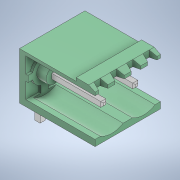
# Autodesk Inventor part: plugin_maleblock
Saved by Autodesk Inventor 2020 (Build 240168000, 168)
## iProperties
Created: 2019-08-19
Part Number: plugin_maleblock
Material: Generic
Document SubType Name: Modeling
Designer: SENSE IT OUT
Density: 1 g/cm^3
Appearance: Default
Mass: 0.267438 g
Surface Area: 8.31838 cm^2
Volume: 0.267438 cm^3
Author: SENSE IT OUT
Autodesk Inventor part; units mm, degrees
ref_plane "YZ Plane" through (0, 0, 0) normal (1, 0, 0) x (0, 1, 0)
ref_plane "XZ Plane" through (0, 0, 0) normal (0, 1, 0) x (-1, 0, 0)
ref_plane "XY Plane" through (0, 0, 0) normal (0, 0, 1) x (1, 0, 0)
sketch "Sketch1" plane through (0, 0, 0) normal (0, 0, 1) x (1, 0, 0)
  line L0 (0, 0) -> (12, 0)
  line L1 (9, 7.5) -> (0, 7.5)
  line L2 (0, 7.5) -> (0, 0)
  line L3 (1, 1) -> (11, 1)
  line L4 (1, 6.5) -> (1, 1)
  line L5 (11, 1) -> (12, 1)
  line L6 (12, 1) -> (12, 0)
  line L7 (12, 7.5) -> (12, 7)
  line L8 (12, 7) -> (1, 7)
  line L9 (1, 6.5) -> (1, 7)
  line L10 (11, 8) -> (9, 8)
  line L11 (9, 8) -> (9, 7.5)
  line L12 (12, 7.5) -> (11, 8)
  dimension "d0" = 7.5
  dimension "d1" = 1
  dimension "d3" = 10
  dimension "d4" = 1
  dimension "d5" = 1
  dimension "d6" = 0.5
  dimension "d7" = 11
  dimension "d10" = 0.5
  dimension "d11" = 11
  dimension "d12" = 0.5
  dimension "d14" = 1
  dimension "d15" = 3
  dimension "d16" = 1
  constraints: 26 end point, 4 perpendicular, 1 horizontal, 1 parallel, 1 vertical
  measures "d0" distance between parallel lines of L0 L1
  measures "d1" distance between parallel lines of L2 L4
  measures "d3" distance of L3.start L3.end
  measures "d4" distance of L3.end L5.end
  measures "d5" distance of L5.end L0.end
  measures "d6" distance of L7.start L7.end
  measures "d7" distance of L7.end L8.end
  measures "d10" distance of L10.end L1.start
  measures "d11" distance between parallel lines of L4 L6
  measures "d12" distance from line of L8 L12.start
  measures "d14" distance from line of L7 L10.start
  measures "d15" distance between parallel lines of L7 L11
  measures "d16" distance between parallel lines of L8 L10
extrude "Extrusion1" add sketch "Sketch1" along normal blind 10.4
sketch "Sketch2" plane through (1, 1, 0) normal (1, 0, 0) x (0, 0, -1)
  circle A0 centre (-7.74, 3) radius 1.27
  circle A1 centre (-2.66, 3) radius 1.27
  line L0 (0, 0) -> (0, 6) projected
  line L1 (0, 0) -> (-10.4, 0) projected
  circle A2 centre (-7.74, 3) radius 2
  circle A3 centre (-2.66, 3) radius 2
  line L2 (-10.4, 0) -> (-10.4, 6) projected
  line L3 (0, 6) -> (-10.4, 6) projected
  line L4 (-7.14, 0) -> (-7.14, 1.0921)
  line L5 (-7.14, 4.9079) -> (-7.14, 6)
  line L6 (-8.34, 6) -> (-8.34, 4.9079)
  line L7 (-8.34, 1.0921) -> (-8.34, 0)
  line L8 (-2.06, 0) -> (-2.06, 1.0921)
  line L9 (-2.06, 4.9079) -> (-2.06, 6)
  line L10 (-3.26, 6) -> (-3.26, 4.9079)
  line L11 (-3.26, 1.0921) -> (-3.26, 0)
  line L12 (-0.7235, 3.5) -> (0, 3.5)
  line L13 (0, 2.5) -> (-0.7235, 2.5)
  line L14 (-5.8035, 3.5) -> (-4.5965, 3.5)
  line L15 (-4.5965, 2.5) -> (-5.8035, 2.5)
  line L16 (-9.6765, 2.5) -> (-10.4, 2.5)
  line L17 (-10.4, 3.5) -> (-9.6765, 3.5)
  point P0 (0, -1)
  dimension "d25" = 4
  dimension "d26" = 4
  dimension "d19" = 5.08
  dimension "d20" = 2.66
  dimension "d21" = 0
  dimension "d22" = 3
  dimension "d23" = 2.54
  dimension "d24" = 2.54
  constraints: 28 end point, 12 perpendicular, 10 point on line, 9 parallel, 3 horizontal, 2 centre point, 2 coincident, 20 other
  measures "d19" distance of A1.centre A0.centre
  measures "d20" distance from line of L0 A1.centre
  measures "d21" vertical distance of A0.centre A1.centre
  measures "d22" distance from line of L1 A1.centre
  measures "d23" diameter of A0
  measures "d24" diameter of A1
extrude "Extrusion2" add sketch "Sketch2" along normal blind 0.35 contours L13 A3 L12 L0 | L1 L11 A3 L8 | A3 | L1 L7 A2 L4 | L9 A3 L10 L3 | A2 | L15 A2 L14 A3 | L5 A2 L6 L3 | L2 L17 A2 L16
sketch "Sketch3" plane through (1.35, 1, 0) normal (1, 0, 0) x (0, 0, -1)
  circle A0 centre (-7.74, 3) radius 1.27 projected
  circle A1 centre (-7.74, 3) radius 1.27
  circle A2 centre (-7.74, 3) radius 2
  circle A3 centre (-2.66, 3) radius 1.27 projected
  circle A4 centre (-2.66, 3) radius 1.27
  circle A5 centre (-2.66, 3) radius 2
  circle A6 centre (-7.74, 3) radius 1.27
  circle A7 centre (-7.74, 3) radius 0.75
  circle A8 centre (-2.66, 3) radius 1.27
  circle A9 centre (-2.66, 3) radius 0.75
  point P0 (0, -1)
  dimension "d49" = 1.5
  dimension "d50" = 1.5
  constraints: 8 centre point, 8 coincident, 1 concentric
  measures "d49" diameter of A7
  measures "d50" diameter of A9
extrude "Extrusion3" add sketch "Sketch3" along normal blind 1.5 contours A0 | A3 | A7 | A9
sketch "Sketch5" plane through (2.85, 4, 7.74) normal (1, 0, 0) x (0, 0, -1)
  line L0 (4.68, 0.4) -> (5.48, 0.4)
  line L1 (5.48, 0.4) -> (5.48, -0.4)
  line L2 (5.48, -0.4) -> (4.68, -0.4)
  line L3 (4.68, -0.4) -> (4.68, 0.4)
  line L4 (-0.4, 0.4) -> (0.4, 0.4)
  line L5 (0.4, 0.4) -> (0.4, -0.4)
  line L6 (0.4, -0.4) -> (-0.4, -0.4)
  line L7 (-0.4, -0.4) -> (-0.4, 0.4)
  circle A0 centre (5.08, 0) radius 1.27 projected
  circle A1 centre (0, 0) radius 1.27 projected
  point P0 (7.74, -4)
  dimension "d51" = 0.4
  dimension "d52" = 0.8
  dimension "d53" = 0.8
  dimension "d54" = 0.4
  dimension "d55" = 0.8
  dimension "d56" = 0.8
  dimension "d57" = 0.4
  constraints: 16 end point, 4 parallel, 2 horizontal, 2 perpendicular, 1 point on line
  measures "d51" distance from line of A0.centre L0
  measures "d52" distance of L0.start L0.end
  measures "d53" distance of L2.end L0.start
  measures "d54" distance from line of A0.centre L3
  measures "d55" distance of L4.start L4.end
  measures "d56" distance of L6.end L4.start
  measures "d57" distance from line of A1.centre L7
extrude "Extrusion5" add sketch "Sketch5" along normal blind 8 contours L0 L1 L2 L3 | L4 L5 L6 L7
chamfer "Chamfer2" distance 0.2 angle 45 8 edges at (10.85, 4.4, 7.74) (10.85, 4.4, 2.66) (10.85, 4, 2.26) (10.85, 4, 3.06) (10.85, 3.6, 2.66) (10.85, 4, 8.14) (10.85, 4, 7.34) (10.85, 3.6, 7.74)
sketch "Sketch6" plane through (9, 8, 0) normal (0, 1, 0) x (1, 0, 0)
  line L0 (3, 0) -> (3, -10.4) projected
  line L1 (2, 0) -> (2, -10.4) projected
  line L2 (3, -0.55) -> (2, -0.55)
  line L3 (2, -0.55) -> (2, -2.05)
  line L4 (2, -2.05) -> (3, -2.05)
  line L5 (3, -2.05) -> (3, -0.55)
  line L6 (3, -0.55) -> (2, -0.8)
  line L7 (3, -2.05) -> (2, -1.8)
  line L8 (3, 0) -> (2, 0) projected
  point P0 (-9, 0)
  point P1 (2, -1.8)
  point P2 (3, -2.05)
  dimension "d69" = 1.5
  dimension "d70" = 1
  dimension "d71" = 0.25
  dimension "d72" = 0.55
  constraints: 12 end point, 4 point on line, 2 parallel, 1 horizontal, 1 perpendicular
  measures "d69" distance between parallel lines of L4 L2
  measures "d70" distance of L7.end L6.end
  measures "d71" distance from line of L2 L6.end
  measures "d72" distance between parallel lines of L8 L2
extrude "Extrusion6" cut sketch "Sketch6" against normal blind 5 contours L0 L7 L1 L6
pattern_linear "Rectangular Pattern1" count 4 spacing 2.6 along (0, 0, 1) of "Extrusion6"
sketch "Sketch7" plane through (12, 0, 0) normal (1, 0, 0) x (0, 0, -1)
  circle A0 centre (-7.74, 4) radius 1.27 projected
  arc A1 (-9.5428, 1) -> (-5.9372, 1) centre (-7.74, 4) ccw
  arc A2 (-4.4628, 1) -> (-0.8572, 1) centre (-2.66, 4) ccw
  circle A3 centre (-2.66, 4) radius 1.27 projected
  line L0 (0, 1) -> (-10.4, 1) projected
  line L1 (-5.9372, 1) -> (-4.4628, 1)
  line L2 (-8.34, 1) -> (-10.4, 1) projected
  line L3 (-9.5428, 1) -> (-10.4, 1)
  line L4 (-10.4, 1) -> (0, 1)
  point P0 (0, 0)
  dimension "d78" = 7
  dimension "d79" = 7
  constraints: 6 end point, 4 point on circle, 4 point on line, 2 centre point, 2 collinear, 1 coincident, 1 concentric
  measures "d78" diameter of A1
  measures "d79" diameter of A2
extrude "Extrusion7" cut sketch "Sketch7" against normal blind 10.65 contours L0 A1 | L0 A2
sketch "Sketch8" plane through (0, 0, 0) normal (0, -1, 0) x (1, 0, 0)
  line L0 (1, 2.26) -> (-0.413, 2.26)
  line L1 (-0.413, 2.26) -> (-0.413, 3.06)
  line L2 (-0.413, 3.06) -> (1, 3.06)
  line L3 (1, 3.06) -> (1, 2.26)
  line L4 (1, 7.34) -> (-0.9223, 7.34)
  line L5 (-0.9223, 7.34) -> (-0.9223, 8.14)
  line L6 (-0.9223, 8.14) -> (1, 8.14)
  line L7 (1, 8.14) -> (1, 7.34)
  line L8 (0, 0) -> (0, 10.4) projected
  line L9 (0, 0) -> (12, 0) projected
  line L10 (0, 10.4) -> (12, 10.4) projected
  line L11 (2.85, 8.14) -> (10.65, 8.14) projected
  line L12 (2.85, 2.26) -> (10.65, 2.26) projected
  point P0 (1, 10.4)
  dimension "d83" = 1
  dimension "d84" = 0.8
  dimension "d85" = 0.8
  dimension "d86" = 2.26
  dimension "d87" = 2.26
  dimension "d88" = 2.26
  dimension "d89" = 2.26
  constraints: 16 end point, 4 parallel, 2 horizontal, 1 perpendicular
  measures "d83" distance between parallel lines of L8 L7
  measures "d84" distance between parallel lines of L2 L0
  measures "d85" distance between parallel lines of L6 L4
  measures "d86" distance between parallel lines of L9 L0
  measures "d87" distance between parallel lines of L6 L10
  measures "d88" distance from line of point (1, 10.4) L11
  measures "d89" distance between parallel lines of L9 L12
extrude "Extrusion8" cut sketch "Sketch8" against normal blind 4.5
sketch "Sketch10" plane through (1, 0, 2.26) normal (-1, 0, 0) x (0, 0, 1)
  line L0 (0, 4.4) -> (0.8, 4.4)
  line L1 (0.8, 4.4) -> (0.8, -3.6)
  line L2 (0.8, -3.6) -> (0, -3.6)
  line L3 (0, -3.6) -> (0, 4.4)
  line L4 (5.08, 4.4) -> (5.88, 4.4)
  line L5 (5.88, 4.4) -> (5.88, -3.6)
  line L6 (5.88, -3.6) -> (5.08, -3.6)
  line L7 (5.08, -3.6) -> (5.08, 4.4)
  line L8 (0.8, 4.5) -> (0.8, 0) projected
  line L9 (5.08, 0) -> (5.08, 4.5) projected
  line L10 (0, 4.5) -> (0.8, 4.5) projected
  arc A0 (0.8, 2.7946) -> (0, 2.7946) centre (0.4, 4) ccw projected
  arc A1 (5.88, 2.7946) -> (5.08, 2.7946) centre (5.48, 4) ccw projected
  point P0 (-2.26, 0)
  dimension "d92" = 0.8
  dimension "d93" = 0.8
  dimension "d96" = 8
  dimension "d101" = 0.4
  dimension "d102" = 0.4
  dimension "d103" = 0.4
  dimension "d106" = 8
  constraints: 16 end point, 4 parallel, 2 horizontal, 2 perpendicular, 1 point on line
  measures "d92" distance of L5.end L6.end
  measures "d93" distance of L1.end L2.end
  measures "d96" distance of L2.end L0.start
  measures "d101" distance from line of L7 A1.centre
  measures "d102" distance from line of L0 A0.centre
  measures "d103" distance from line of L3 A0.centre
  measures "d106" distance of L6.end L4.start
extrude "Extrusion9" add sketch "Sketch10" along normal blind 0.8 contours L0 L1 L2 L3 | L4 L5 L6 L7
sketch "Sketch11" plane through (1, 1, 10.4) normal (1, 0, 0) x (0, 0, -1)
  point P0 (10.4, -1)
chamfer "Chamfer3" distance 0.2 angle 45 8 edges at (0.6, -3.6, 8.14) (0.2, -3.6, 7.74) (0.6, -3.6, 7.34) (1, -3.6, 7.74) (0.2, -3.6, 2.66) (0.6, -3.6, 2.26) (0.6, -3.6, 3.06) (1, -3.6, 2.66)
fillet "Fillet1" radius 0.2 2 edges at (0.2, 4.4, 2.66) (0.2, 4.4, 7.74)
sketch "Sketch12" plane through (0, 0, 0) normal (-1, 0, 0) x (0, 0, 1)
  line L0 (1.91, 7) -> (3.41, 7)
  line L1 (3.41, 7) -> (3.41, 0)
  line L2 (1.91, 0) -> (1.91, 7)
  line L3 (6.99, 7) -> (8.49, 7)
  line L4 (8.49, 7) -> (8.49, 0)
  line L5 (6.99, 0) -> (6.99, 7)
  line L6 (8.14, 0) -> (10.4, 0) projected
  line L7 (3.06, 0) -> (7.34, 0) projected
  line L8 (0, 7.5) -> (10.4, 7.5) projected
  line L9 (3.06, -3.4) -> (3.06, 0) projected
  line L10 (8.14, 4.5) -> (8.14, 0) projected
  line L11 (2.26, 0) -> (2.26, 4.5) projected
  line L12 (0, 0) -> (2.26, 0) projected
  line L13 (2.26, 0) -> (2.26, -3.4) projected
  line L14 (2.26, 4.4) -> (3.06, 4.4) projected
  line L15 (2.26, 0) -> (3.06, 0)
  line L16 (3.06, 0) -> (3.06, 4.4)
  line L17 (3.06, 4.4) -> (2.26, 4.4)
  line L18 (2.26, 4.4) -> (2.26, 0)
  line L19 (7.34, 4.4) -> (8.14, 4.4) projected
  line L20 (8.14, 0) -> (8.14, 4.4)
  line L21 (8.14, 4.4) -> (7.34, 4.4)
  line L22 (7.34, 4.4) -> (7.34, 0)
  line L23 (3.41, 0) -> (3.06, 0)
  line L24 (2.26, 0) -> (1.91, 0)
  line L25 (8.49, 0) -> (8.14, 0)
  line L26 (7.34, 0) -> (6.99, 0)
  point P0 (3.41, 0)
  dimension "d111" = 1.5
  dimension "d112" = 1.5
  dimension "d115" = 0.5
  dimension "d116" = 0.5
  dimension "d117" = 0.35
  dimension "d118" = 0.35
  constraints: 35 end point, 9 parallel, 3 horizontal, 3 perpendicular
  measures "d111" distance between parallel lines of L1 L2
  measures "d112" distance between parallel lines of L4 L5
  measures "d115" distance between parallel lines of L8 L0
  measures "d116" distance between parallel lines of L3 L8
  measures "d117" distance between parallel lines of L9 L1
  measures "d118" distance between parallel lines of L10 L4
extrude "Extrusion10" cut sketch "Sketch12" against normal blind 0.1 contours L5 L3 L4 L6 L10 L19 L22 L7 | L0 L1 L7 L16 L14 L11 L12 L2
sketch "Sketch13" plane through (0, 0, 0) normal (0, -1, 0) x (1, 0, 0)
  line L0 (0.1, 1.91) -> (0, 1.91) projected
  line L1 (0.1, 1.91) -> (1.35, 1.91)
  line L2 (1.35, 1.91) -> (1.35, 3.41)
  line L3 (1.35, 3.41) -> (0.1, 3.41)
  line L4 (0.1, 3.41) -> (0.1, 1.91)
  line L5 (0.1, 6.99) -> (0.1, 8.49) projected
  line L6 (0.1, 6.99) -> (1.35, 6.99)
  line L7 (1.35, 6.99) -> (1.35, 8.49)
  line L8 (1.35, 8.49) -> (0.1, 8.49)
  line L9 (0.1, 8.49) -> (0.1, 6.99)
  line L10 (1, 7.34) -> (1, 8.14) projected
  line L11 (0, 3.41) -> (0.1, 3.41) projected
  line L12 (1, 2.26) -> (1, 3.06) projected
  line L13 (0.1, 8.14) -> (1, 8.14) projected
  line L14 (0.4, 7.34) -> (1, 7.34) projected
  line L15 (0.1, 8.14) -> (1, 8.14)
  line L16 (1, 8.14) -> (1, 7.34)
  line L17 (1, 7.34) -> (0.1, 7.34)
  line L18 (0.1, 7.34) -> (0.1, 8.14)
  line L19 (0.1, 3.06) -> (0.1, 2.26) projected
  line L20 (0.1, 3.06) -> (1, 3.06)
  line L21 (1, 3.06) -> (1, 2.26)
  line L22 (1, 2.26) -> (0.1, 2.26)
  line L23 (0.1, 2.26) -> (0.1, 3.06)
  point P0 (0, 0)
  dimension "d130" = 0.35
  dimension "d131" = 0
  dimension "d132" = 0.35
  constraints: 32 end point, 8 parallel, 4 horizontal, 4 perpendicular
  measures "d130" distance between parallel lines of L7 L10
  measures "d131" distance between parallel lines of L3 L11
  measures "d132" distance between parallel lines of L2 L12
extrude "Extrusion11" cut sketch "Sketch13" against normal blind 0.1 contours L4 L22 L12 L20 L3 L2 L1 | L5 L17 L14 L10 L13 L8 L7 L6
body "Solid1"
